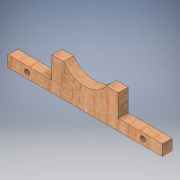
# Autodesk Inventor part: Soporte para Motor 2
Saved by Autodesk Inventor 2016 SP2 (Build 200236200, 236)
## iProperties
Created: 2017-06-02
Part Number: Soporte para Motor 2
Material: Abedul
Document SubType Name: Modeling
Designer: ssant
Density: 0.512 g/cm^3
Appearance: Abedul - Natural brillo medio
Author: ssant
Autodesk Inventor part; units mm, degrees
ref_plane "YZ Plane" through (0, 0, 0) normal (1, 0, 0) x (0, 1, 0)
ref_plane "XZ Plane" through (0, 0, 0) normal (0, 1, 0) x (-1, 0, 0)
ref_plane "XY Plane" through (0, 0, 0) normal (0, 0, 1) x (1, 0, 0)
sketch "Boceto3" plane through (0, 0, 0) normal (0, 0, 1) x (1, 0, 0)
  line L0 (-30, 8) -> (-30, -12)
  line L1 (-30, -22) -> (30, -22)
  line L2 (30, -12) -> (30, 8)
  arc A0 (-19.4936, 8) -> (19.4936, 8) centre (0, 22) ccw
  line L3 (-30, 8) -> (-19.4936, 8)
  line L4 (19.4936, 8) -> (30, 8)
  line L5 (-30, -22) -> (-70, -22)
  line L6 (-70, -22) -> (-70, -12)
  line L7 (-70, -12) -> (-30, -12)
  line L8 (30, -22) -> (70, -22)
  line L9 (70, -22) -> (70, -12)
  line L10 (70, -12) -> (30, -12)
  point P0 (0, 0)
  point P1 (0, -22)
  point P2 (30, 0)
  dimension "d16" = 60
  dimension "d38" = 24
  dimension "d39" = 10.5064
  dimension "d40" = 10.5064
  dimension "d41" = 30
  dimension "d42" = 30
  dimension "d43" = 22
  dimension "d44" = 40
  dimension "d45" = 10
  dimension "d46" = 40
  dimension "d47" = 10
  constraints: 22 end point, 7 perpendicular, 3 horizontal, 2 point on circle, 1 centre point, 1 horizontal alignment, 1 midpoint, 1 point on line, 1 vertical, 1 vertical alignment
  measures "d16" distance of L1.start L1.end
  measures "d38" radius of A0
  measures "d39" distance of L4.start L2.end
  measures "d40" distance of L0.start L3.end
  measures "d41" distance from line of L2 A0.centre
  measures "d42" distance between parallel lines of L1 L4
  measures "d43" distance from line of L1 point (0, 0)
  measures "d44" distance of L1.start L5.end
  measures "d45" distance of L5.end L6.end
  measures "d46" distance of L1.end L8.end
  measures "d47" distance of L8.end L9.end
extrude "Extrusión2" add sketch "Boceto3" along normal blind 9
sketch "Boceto5" plane through (0, 0, 9) normal (0, 0, 1) x (1, 0, 0)
  line L0 (-70, -22) -> (70, -22) projected
  line L1 (70, -22) -> (70, -12) projected
  line L2 (70, -12) -> (30, -12) projected
  line L3 (30, -12) -> (30, 8) projected
  line L4 (30, 8) -> (19.4936, 8) projected
  arc A0 (-19.4936, 8) -> (19.4936, 8) centre (0, 22) ccw projected
  line L5 (-19.4936, 8) -> (-30, 8) projected
  line L6 (-30, 8) -> (-30, -12) projected
  line L7 (-30, -12) -> (-70, -12) projected
  line L8 (-70, -12) -> (-70, -22) projected
  point P0 (0, 0)
  point P1 (-52.5, -17)
  point P2 (52.5, -17)
  dimension "d55" = 5
  dimension "d56" = 17.5
  dimension "d57" = 5
  dimension "d58" = 17.5
  measures "d55" distance from line of L2 point (52.5, -17)
  measures "d56" distance from line of L1 point (52.5, -17)
  measures "d57" distance from line of L7 point (-52.5, -17)
  measures "d58" distance from line of L8 point (-52.5, -17)
hole "Agujero2" at (-52.5, -17, 9) at (52.5, -17, 9) direction (0, 0, -1) diameter 5 depth 10 tip angle 118
sketch "Boceto6" plane through (-70, -22, 0) normal (0, -1, 0) x (1, 0, 0)
  line L0 (0, 0) -> (140, 0) projected
  line L1 (140, 0) -> (140, 9) projected
  line L2 (0, 9) -> (140, 9) projected
  line L3 (0, 0) -> (0, 9) projected
  line L4 (40, 0) -> (40, 9) projected
  line L5 (100, 0) -> (100, 9) projected
  point P0 (70, 0)
  point P1 (47.5, 4.5)
  point P2 (92.5, 4.5)
  dimension "d67" = 47.5
  dimension "d68" = 47.5
  dimension "d69" = 4.5
  dimension "d70" = 4.5
  measures "d67" distance from line of L3 point (47.5, 4.5)
  measures "d68" distance from line of L1 point (92.5, 4.5)
  measures "d69" distance from line of L2 point (92.5, 4.5)
  measures "d70" distance from line of L2 point (47.5, 4.5)
hole "Agujero3" at (-22.5, -22, 4.5) at (22.5, -22, 4.5) direction (0, 1, 0) diameter 5 depth 20 tip angle 118
